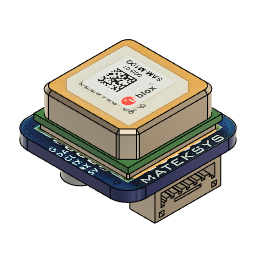
Mateksys M10Q-5883 v6 (Autodesk Fusion 360 design; units mm, degrees)
Autodesk Fusion 360 part; units mm, degrees
sketch "Sketch2" plane through (0, 0, 0) normal (0, 0, 1) x (1, 0, 0)
  line L0 (10, -10) -> (-10, -10)
  line L1 (-10, -10) -> (-10, 10)
  line L2 (-10, 10) -> (10, 10)
  line L3 (10, 10) -> (10, -10)
  line L4 (10, -10) -> (-10, 10) construction
  line L5 (-10, -10) -> (10, 10) construction
  dimension "d1" = 20
  dimension "d2" = 20
  constraint horizontal L0
  constraint perpendicular L0 L1
  constraint parallel L0 L2
  constraint parallel L1 L3
  constraint coincident L4 origin
  constraint coincident L5 origin
  measures "d1" distance of L1.end L2.end
  measures "d2" distance of L0.end L1.end
extrude "Extrude1" add sketch "Sketch2" against normal blind 1.75 makes body 1
sketch "Sketch3" plane through (-10, 0, 0) normal (-1, 0, 0) x (0, -1, 0)
  line L0 (10, 0) -> (-10, 0)
  line L1 (-10, 0) -> (-10, -1.75)
  line L2 (-10, -1.75) -> (10, -1.75)
  line L3 (10, -1.75) -> (10, 0)
  line L4 (-5.6474, -1.75) -> (5.4445, -1.75)
  line L5 (5.4445, -1.75) -> (5.4445, -6.1546)
  line L6 (5.4445, -6.1546) -> (-5.6474, -6.1546)
  line L7 (-5.6474, -6.1546) -> (-5.6474, -1.75)
  constraint horizontal L4
  constraint vertical L5
  constraint horizontal L6
  constraint vertical L7
  constraint coincident L2 L4.start
extrude "Extrude2" add sketch "Sketch3" against normal blind 4.25 separate body contours L2 L4 L5 L6 L7 makes body 2
sketch "Sketch4" plane through (0, 0, -1.75) normal (0, 0, -1) x (1, 0, 0)
  line L0 (-10, -10) -> (10, -10)
  line L1 (10, -10) -> (10, 10)
  line L2 (10, 10) -> (-10, 10)
  line L3 (-10, 10) -> (-10, -10)
  circle A0 centre (-0.758, 7.2611) radius 2.3938
extrude "Extrude3" add sketch "Sketch4" along normal blind 1.745 contours A0 bodies 1
sketch "Sketch5" plane through (0, 0, -1.75) normal (0, 0, -1) x (1, 0, 0)
  circle A0 centre (-0.758, 7.2611) radius 2.3938
  line L0 (-10, -10) -> (10, -10)
  line L1 (10, -10) -> (10, 10)
  line L2 (10, 10) -> (-10, 10)
  line L3 (-10, 10) -> (-10, -10)
  line L4 (-5.3613, 8.7229) -> (-4.3429, 8.7229)
  line L5 (-4.3429, 8.7229) -> (-4.3429, 6.464)
  line L6 (-4.3429, 6.464) -> (-5.3613, 6.464)
  line L7 (-5.3613, 6.464) -> (-5.3613, 8.7229)
  line L8 (1.3278, 3.0969) -> (2.4368, 3.0969)
  line L9 (2.4368, 3.0969) -> (2.4368, 0.8543)
  line L10 (2.4368, 0.8543) -> (1.3278, 0.8543)
  line L11 (1.3278, 0.8543) -> (1.3278, 3.0969)
  line L12 (2.8558, 3.0969) -> (3.7676, 3.0969)
  line L13 (3.7676, 3.0969) -> (3.7676, 0.8543)
  line L14 (3.7676, 0.8543) -> (2.8558, 0.8543)
  line L15 (2.8558, 0.8543) -> (2.8558, 3.0969)
  line L16 (-2.147, 2.7766) -> (0.8103, 2.7766)
  line L17 (0.8103, 2.7766) -> (0.8103, 1.1747)
  line L18 (0.8103, 1.1747) -> (-2.147, 1.1747)
  line L19 (-2.147, 1.1747) -> (-2.147, 2.7766)
  line L20 (2.5847, 6.9907) -> (4.014, 6.9907)
  line L21 (4.014, 6.9907) -> (4.014, 4.4523)
  line L22 (4.014, 4.4523) -> (2.5847, 4.4523)
  line L23 (2.5847, 4.4523) -> (2.5847, 6.9907)
  line L24 (2.5847, 9.4258) -> (4.6888, 9.4258)
  line L25 (4.6888, 9.4258) -> (4.6888, 8.6473)
  line L26 (4.6888, 8.6473) -> (2.5847, 8.6473)
  line L27 (2.5847, 8.6473) -> (2.5847, 9.4258)
  line L28 (-1.5553, -3.4636) -> (1.4867, -3.4636)
  line L29 (1.4867, -3.4636) -> (1.4867, -6.4798)
  line L30 (1.4867, -6.4798) -> (-1.5553, -6.4798)
  line L31 (-1.5553, -6.4798) -> (-1.5553, -3.4636)
  line L32 (1.9507, -7.2532) -> (3.6522, -7.2532)
  line L33 (3.6522, -7.2532) -> (3.6522, -8.0524)
  line L34 (3.6522, -8.0524) -> (1.9507, -8.0524)
  line L35 (1.9507, -8.0524) -> (1.9507, -7.2532)
  line L36 (1.9507, -8.8516) -> (3.6522, -8.8516)
  line L37 (3.6522, -8.8516) -> (3.6522, -9.7281)
  line L38 (3.6522, -9.7281) -> (1.9507, -9.7281)
  line L39 (1.9507, -9.7281) -> (1.9507, -8.8516)
  line L40 (-1.6327, -8.8516) -> (0.1254, -8.8516)
  line L41 (0.1254, -8.8516) -> (0.1254, -9.7281)
  line L42 (0.1254, -9.7281) -> (-1.6327, -9.7281)
  line L43 (-1.6327, -9.7281) -> (-1.6327, -8.8516)
  line L44 (-4.5598, -7.5897) -> (-2.7838, -7.5897)
  line L45 (-2.7838, -7.5897) -> (-2.7838, -8.3846)
  line L46 (-2.7838, -8.3846) -> (-4.5598, -8.3846)
  line L47 (-4.5598, -8.3846) -> (-4.5598, -7.5897)
  line L48 (-4.5598, -6.1689) -> (-2.7838, -6.1689)
  line L49 (-2.7838, -6.1689) -> (-2.7838, -6.9131)
  line L50 (-2.7838, -6.9131) -> (-4.5598, -6.9131)
  line L51 (-4.5598, -6.9131) -> (-4.5598, -6.1689)
  line L52 (-4.5598, -4.6804) -> (-2.7838, -4.6804)
  line L53 (-2.7838, -4.6804) -> (-2.7838, -5.4754)
  line L54 (-2.7838, -5.4754) -> (-4.5598, -5.4754)
  line L55 (-4.5598, -5.4754) -> (-4.5598, -4.6804)
  line L56 (-3.6718, -0.4539) -> (-2.2377, -0.4539)
  line L57 (-2.2377, -0.4539) -> (-2.2377, -3.0706)
  line L58 (-2.2377, -3.0706) -> (-3.6718, -3.0706)
  line L59 (-3.6718, -3.0706) -> (-3.6718, -0.4539)
  line L60 (2.7373, -4.3628) -> (3.6095, -4.3628)
  line L61 (3.6095, -4.3628) -> (3.6095, -6.1689)
  line L62 (3.6095, -6.1689) -> (2.7373, -6.1689)
  line L63 (2.7373, -6.1689) -> (2.7373, -4.3628)
  line L64 (4.2045, -4.5697) -> (5.025, -4.5697)
  line L65 (5.025, -4.5697) -> (5.025, -6.1689)
  line L66 (5.025, -6.1689) -> (4.2045, -6.1689)
  line L67 (4.2045, -6.1689) -> (4.2045, -4.5697)
  line L68 (-1.6553, -0.4628) -> (0.2255, -0.4628)
  line L69 (0.2255, -0.4628) -> (0.2255, -1.315)
  line L70 (0.2255, -1.315) -> (-1.6553, -1.315)
  line L71 (-1.6553, -1.315) -> (-1.6553, -0.4628)
  constraint horizontal L4
  constraint vertical L5
  constraint horizontal L6
  constraint vertical L7
  constraint horizontal L8
  constraint vertical L9
  constraint horizontal L10
  constraint vertical L11
  constraint horizontal L12
  constraint vertical L13
  constraint horizontal L14
  constraint vertical L15
  constraint horizontal L16
  constraint vertical L17
  constraint horizontal L18
  constraint vertical L19
  constraint horizontal L20
  constraint vertical L21
  constraint horizontal L22
  constraint vertical L23
  constraint horizontal L24
  constraint vertical L25
  constraint horizontal L26
  constraint vertical L27
  constraint horizontal L28
  constraint vertical L29
  constraint horizontal L30
  constraint vertical L31
  constraint horizontal L32
  constraint vertical L33
  constraint horizontal L34
  constraint vertical L35
  constraint horizontal L36
  constraint vertical L37
  constraint horizontal L38
  constraint vertical L39
  constraint horizontal L40
  constraint vertical L41
  constraint horizontal L42
  constraint vertical L43
  constraint horizontal L44
  constraint vertical L45
  constraint horizontal L46
  constraint vertical L47
  constraint horizontal L48
  constraint vertical L49
  constraint horizontal L50
  constraint vertical L51
  constraint horizontal L52
  constraint vertical L53
  constraint horizontal L54
  constraint vertical L55
  constraint horizontal L56
  constraint vertical L57
  constraint horizontal L58
  constraint vertical L59
  constraint horizontal L60
  constraint vertical L61
  constraint horizontal L62
  constraint vertical L63
  constraint horizontal L64
  constraint vertical L65
  constraint horizontal L66
  constraint vertical L67
  constraint horizontal L68
  constraint vertical L69
  constraint horizontal L70
  constraint vertical L71
extrude "Extrude4" add sketch "Sketch5" along normal blind 0.304 contours L4 L5 L6 L7 | L8 L9 L10 L11 | L12 L13 L14 L15 | L20 L21 L22 L23 | L24 L25 L26 L27 | L32 L33 L34 L35 | L36 L37 L38 L39 | L40 L41 L42 L43 | L44 L45 L46 L47 | L48 L49 L50 L51 | L52 L53 L54 L55 | L56 L57 L58 L59 | L60 L61 L62 L63 | L64 L65 L66 L67 | L68 L69 L70 L71 bodies 1
extrude "Extrude5" add sketch "Sketch5" along normal blind 0.555 contours L16 L17 L18 L19 | L28 L29 L30 L31 bodies 1
fillet "Fillet1" radius 3 4 edges at (10, -10, -0.875) (10, 10, -0.875) (-10, -10, -0.875) (-10, 10, -0.875) on bodies 1
sketch "Sketch8" plane through (0, 0, 0) normal (1, 0, 0) x (0, 1, 0)
  line L0 (-7, 0) -> (7, 0)
  line L1 (0, 0) -> (7.8235, 0)
  line L2 (0, 0) -> (0, 1.2209) construction
  line L3 (0, 0) -> (-7.8235, 0)
  constraint coincident L1.start L2.start
  constraint parallel L0 L1
  constraint perpendicular L1 L2
  constraint symmetric L1.start L2 L3.start
  constraint symmetric L1.end L2 L3.end
sketch "Sketch9" plane through (0, 0, 0) normal (0, 0, 1) x (1, 0, 0)
  line L0 (7.5, -7.5) -> (-7.5, -7.5)
  line L1 (-7.5, -7.5) -> (-7.5, 7.5)
  line L2 (-7.5, 7.5) -> (7.5, 7.5)
  line L3 (7.5, 7.5) -> (7.5, -7.5)
  line L4 (7.5, -7.5) -> (-7.5, 7.5) construction
  line L5 (-7.5, -7.5) -> (7.5, 7.5) construction
  dimension "d19" = 15
  dimension "d20" = 15
  constraint horizontal L0
  constraint perpendicular L0 L1
  constraint parallel L0 L2
  constraint parallel L1 L3
  constraint coincident L4 origin
  constraint coincident L5 origin
  measures "d19" distance of L1.end L2.end
  measures "d20" distance of L0.end L1.end
extrude "Extrude7" add sketch "Sketch9" along normal blind 1.145 separate body makes body 3
sketch "Sketch10" plane through (0, 0, 1.145) normal (0, 0, 1) x (-1, 0, 0)
  line L0 (-7.5, -7.5) -> (7.5, -7.5)
  line L1 (7.5, -7.5) -> (7.5, 7.5)
  line L2 (7.5, 7.5) -> (-7.5, 7.5)
  line L3 (-7.5, 7.5) -> (-7.5, -7.5)
  line L4 (-7.9638, 7.9342) -> (7.9638, 7.9342)
  line L5 (7.9638, 7.9342) -> (7.9638, -7.9342)
  line L6 (7.9638, -7.9342) -> (-7.9638, -7.9342)
  line L7 (-7.9638, -7.9342) -> (-7.9638, 7.9342)
  line L8 (-7.9638, 7.9342) -> (7.9638, -7.9342) construction
  line L9 (7.9638, 7.9342) -> (-7.9638, -7.9342) construction
  constraint horizontal L4
  constraint perpendicular L4 L5
  constraint parallel L4 L6
  constraint parallel L5 L7
  constraint coincident L8 origin
  constraint coincident L9 origin
extrude "Extrude8" add sketch "Sketch10" along normal blind 0.974 separate body contours L0 L1 L2 L3 | L4 L5 L6 L7 makes body 4
sketch "Sketch11" plane through (0, 0, 2.119) normal (0, 0, 1) x (-1, 0, 0)
  line L0 (-7.9638, -7.9342) -> (7.9638, -7.9342)
  line L1 (7.9638, -7.9342) -> (7.9638, 7.9342)
  line L2 (7.9638, 7.9342) -> (-7.9638, 7.9342)
  line L3 (-7.9638, 7.9342) -> (-7.9638, -7.9342)
  line L4 (7.5612, 7.5931) -> (-7.5612, 7.5931)
  line L5 (-7.5612, 7.5931) -> (-7.5612, -7.5931)
  line L6 (-7.5612, -7.5931) -> (7.5612, -7.5931)
  line L7 (7.5612, -7.5931) -> (7.5612, 7.5931)
  line L8 (7.5612, 7.5931) -> (-7.5612, -7.5931) construction
  line L9 (-7.5612, 7.5931) -> (7.5612, -7.5931) construction
  constraint horizontal L4
  constraint perpendicular L4 L5
  constraint parallel L4 L6
  constraint parallel L5 L7
  constraint coincident L8 origin
  constraint coincident L9 origin
extrude "Extrude9" add sketch "Sketch11" along normal blind 4.086 separate body contours L4 L5 L6 L7 makes body 5
fillet "Fillet2" radius 1.75 4 edges at (7.5612, -7.5931, 4.162) (7.5612, 7.5931, 4.162) (-7.5612, -7.5931, 4.162) (-7.5612, 7.5931, 4.162) on bodies 5
sketch "Sketch12" plane through (0, 0, 6.205) normal (0, 0, 1) x (-1, 0, 0)
  arc A0 (5.8112, -7.5931) -> (7.5612, -5.8431) centre (5.8112, -5.8431) ccw
  line L0 (7.5612, -5.8431) -> (7.5612, 5.8431)
  arc A1 (7.5612, 5.8431) -> (5.8112, 7.5931) centre (5.8112, 5.8431) ccw
  line L1 (5.8112, 7.5931) -> (-5.8112, 7.5931)
  arc A2 (-5.8112, 7.5931) -> (-7.5612, 5.8431) centre (-5.8112, 5.8431) ccw
  line L2 (-7.5612, 5.8431) -> (-7.5612, -5.8431)
  arc A3 (-7.5612, -5.8431) -> (-5.8112, -7.5931) centre (-5.8112, -5.8431) ccw
  line L3 (-5.8112, -7.5931) -> (5.8112, -7.5931)
  line L4 (-5.8112, 7.5931) -> (-7.5612, 5.8431)
  constraint coincident L1.end A2.start
  constraint coincident A2.end L2.start
extrude "Extrude10" cut sketch "Sketch12" against normal blind 4.086 contours A2 L4 bodies 3 4 1 5
fillet "Fillet3" radius 0.5 2 edges at (5.8112, -7.5931, 4.162) (7.5612, -5.8431, 4.162) on bodies 5
chamfer "Chamfer1" distance 0.5 angle 45 10 edges at (-0.1036, -7.5931, 6.205) (5.7954, -7.555, 6.205) (6.6862, -6.7181, 6.205) (7.5231, -5.8273, 6.205) (7.5612, 0.1036, 6.205) (7.0486, 7.0805, 6.205) (0, 7.5931, 6.205) (-7.0486, 7.0805, 6.205) (-7.5612, 0, 6.205) (-7.0486, -7.0805, 6.205) on bodies 5
sketch "Sketch14" plane through (-10, 0, 0) normal (-1, 0, 0) x (0, -1, 0)
  line L0 (-5.6474, -6.1546) -> (5.4445, -6.1546)
  line L1 (5.4445, -6.1546) -> (5.4445, -1.75)
  line L2 (5.4445, -1.75) -> (-5.6474, -1.75)
  line L3 (-5.6474, -1.75) -> (-5.6474, -6.1546)
  line L4 (-0.1014, -1.75) -> (-0.1014, -6.1546) construction
  line L5 (-0.1014, -2.3405) -> (-4.6247, -2.3405)
  line L6 (-4.6247, -2.3405) -> (-4.6247, -4.4408)
  line L7 (-4.6247, -4.4408) -> (-4.1136, -4.4408)
  line L8 (-4.1136, -4.4408) -> (-4.1136, -3.9523)
  line L9 (-4.1136, -3.9523) -> (-0.1014, -3.9523)
  line L10 (-1.1172, -3.9523) -> (-1.1172, -3.512)
  line L11 (-1.1172, -3.512) -> (-0.3386, -3.512)
  line L12 (-0.3386, -3.512) -> (-0.3386, -3.9523)
  line L13 (-4.9093, -5.0169) -> (-4.1296, -5.0169)
  line L14 (-4.1296, -5.0169) -> (-4.1296, -5.7239)
  line L15 (-4.1296, -5.7239) -> (-4.9093, -5.7239)
  line L16 (-4.9093, -5.7239) -> (-4.9093, -5.0169)
  line L17 (-0.1014, -4.7085) -> (-2.3089, -4.7085)
  line L18 (-2.3089, -4.7085) -> (-2.3089, -4.2823)
  line L19 (-2.3089, -4.2823) -> (-0.1014, -4.2823)
  line L20 (-2.4257, -3.512) -> (-1.6471, -3.512)
  line L21 (-1.6471, -3.512) -> (-1.6471, -3.9523)
  line L22 (-2.4257, -3.9523) -> (-2.4257, -3.512)
  line L23 (-3.7342, -3.512) -> (-2.9556, -3.512)
  line L24 (-2.9556, -3.512) -> (-2.9556, -3.9523)
  line L25 (-3.7342, -3.9523) -> (-3.7342, -3.512)
  line L26 (-1.6471, -3.9523) -> (-2.4257, -3.9523)
  line L27 (-2.9556, -3.9523) -> (-3.7342, -3.9523)
  line L28 (3.5313, -3.512) -> (2.7527, -3.512)
  line L29 (2.7527, -3.512) -> (2.7527, -3.9523)
  line L30 (3.5313, -3.9523) -> (3.5313, -3.512)
  line L31 (1.4442, -3.9523) -> (2.2228, -3.9523)
  line L32 (1.4442, -3.512) -> (1.4442, -3.9523)
  line L33 (2.2228, -3.512) -> (1.4442, -3.512)
  line L34 (2.2228, -3.9523) -> (2.2228, -3.512)
  line L35 (3.9107, -3.9523) -> (-0.1014, -3.9523)
  line L36 (0.1357, -3.512) -> (0.1357, -3.9523)
  line L37 (0.9143, -3.512) -> (0.1357, -3.512)
  line L38 (0.9143, -3.9523) -> (0.9143, -3.512)
  line L39 (3.9107, -4.4408) -> (3.9107, -3.9523)
  line L40 (4.4218, -4.4408) -> (3.9107, -4.4408)
  line L41 (4.4218, -2.3405) -> (4.4218, -4.4408)
  line L42 (-0.1014, -2.3405) -> (4.4218, -2.3405)
  line L43 (2.106, -4.2823) -> (-0.1014, -4.2823)
  line L44 (2.106, -4.7085) -> (2.106, -4.2823)
  line L45 (-0.1014, -4.7085) -> (2.106, -4.7085)
  line L46 (3.9267, -5.0169) -> (3.9267, -5.7239)
  line L47 (4.7064, -5.0169) -> (3.9267, -5.0169)
  line L48 (4.7064, -5.7239) -> (4.7064, -5.0169)
  line L49 (3.9267, -5.7239) -> (4.7064, -5.7239)
  dimension "d36" = -2.617
  dimension "d37" = 0
  constraint midpoint L2 L4.start
  constraint midpoint L0 L4.end
  constraint coincident L4 L5.start
  constraint perpendicular L4 L5
  constraint perpendicular L5 L6
  constraint perpendicular L6 L7
  constraint perpendicular L7 L8
  constraint midpoint L4 L9.end
  constraint coincident L9 L10.start
  constraint perpendicular L9 L10
  constraint perpendicular L10 L11
  constraint coincident L9 L12.end
  constraint perpendicular L9 L12
  constraint horizontal L13
  constraint vertical L14
  constraint horizontal L15
  constraint vertical L16
  constraint coincident L4 L17.start
  constraint perpendicular L4 L17
  constraint perpendicular L17 L18
  constraint coincident L4 L19.end
  constraint perpendicular L4 L19
  constraint perpendicular L22 L26
  constraint perpendicular L25 L27
  constraint horizontal L9
  constraint coincident L8.end L9.start
  constraint symmetric L4 L5.start L42.start
  constraint symmetric L4 L5.end L41.start
  constraint symmetric L4 L6.end L40.start
  constraint symmetric L4 L7.end L39.start
  constraint symmetric L4 L8.end L35.start
  constraint symmetric L4 L9.end L35.end
  constraint symmetric L4 L10.start L38.start
  constraint symmetric L4 L10.end L37.start
  constraint symmetric L4 L11.end L36.start
  constraint symmetric L4 L12.end L36.end
  constraint symmetric L4 L13.start L47.start
  constraint symmetric L4 L13.end L46.start
  constraint symmetric L4 L14.end L46.end
  constraint symmetric L4 L15.end L48.start
  constraint symmetric L4 L17.start L45.start
  constraint symmetric L4 L17.end L44.start
  constraint symmetric L4 L18.end L43.start
  constraint symmetric L4 L19.end L43.end
  constraint symmetric L4 L20.start L33.start
  constraint symmetric L4 L20.end L32.start
  constraint symmetric L4 L21.end L31.start
  constraint symmetric L4 L22.start L31.end
  constraint symmetric L4 L23.start L28.start
  constraint symmetric L4 L23.end L28.end
  constraint symmetric L4 L24.end L29.end
  constraint symmetric L4 L25.start L30.start
extrude "Extrude11" cut sketch "Sketch14" against normal blind 3.268 contours L5 L6 L7 L8 L9 L10 L11 L12 L20 L21 L22 L23 L24 L25 L28 L29 L30 L32 L33 L34 L35 L36 L37 L38 L39 L40 L41 L42 | L13 L14 L15 L16 | L17 L18 L19 L43 L44 L45 | L46 L47 L48 L49 bodies 2
mirror "Mirror2" about plane through (0, 0, 0) normal (1, 0, 0) of bodies 2 makes body 6
fillet "Fillet4" radius 0.25 4 edges at (-7.5, 7.5, 0.5725) (7.5, 7.5, 0.5725) (7.5, -7.5, 0.5725) (-7.5, -7.5, 0.5725) on bodies 3
extrude "Extrude12" add 2 faces at (-8.5833, -1.7472, -6.1546) (8.5833, -1.7472, -6.1546) along direction (0, 0, -1) blind 0.04 on bodies 2 6 bodies 2 6
